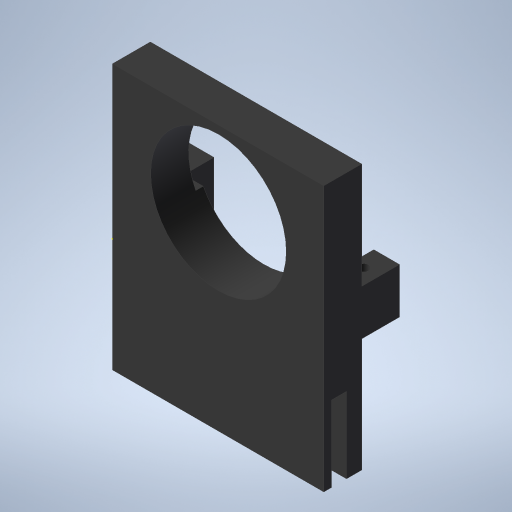
# Autodesk Inventor part: Part8
Saved by Autodesk Inventor 2023.2 (Build 272271030, 271C)
## iProperties
Created: 2024-03-23
Part Number: Part8
Material: Generic
Document SubType Name: Modeling
Designer: ryanv
Density: 1 g/cm^3
Appearance: Default
Author: ryanv
Autodesk Inventor part; units mm, degrees
ref_plane "YZ Plane" through (0, 0, 0) normal (1, 0, 0) x (0, 1, 0)
ref_plane "XZ Plane" through (0, 0, 0) normal (0, 1, 0) x (-1, 0, 0)
ref_plane "XY Plane" through (0, 0, 0) normal (0, 0, 1) x (1, 0, 0)
sketch "Sketch1" plane through (0, 0, 0) normal (0, 0, 1) x (1, 0, 0)
  line L0 (0, 40) -> (55.8, 40)
  line L1 (55.8, 40) -> (55.8, 0)
  line L2 (55.8, 0) -> (0, 0)
  line L3 (0, 0) -> (0, 40)
  dimension "d0" = 55.8
  dimension "d1" = 40
  constraints: 8 end point, 2 parallel, 1 horizontal, 1 perpendicular
  measures "d0" distance of L1.end L2.end
  measures "d1" distance between parallel lines of L2 L0
extrude "Extrusion1" add sketch "Sketch1" along normal blind 20
sketch "Sketch2" plane through (55.8, 0, 0) normal (1, 0, 0) x (0, 0, -1)
  line L0 (0, 40) -> (-20, 40) projected
  line L1 (0, 0) -> (0, 40) projected
  line L2 (-10, 40) -> (0, 40)
  line L3 (0, 40) -> (0, 12)
  line L4 (0, 12) -> (-10, 12)
  line L5 (-10, 12) -> (-10, 40)
  dimension "d4" = 10
  constraints: 8 end point, 2 parallel, 1 horizontal, 1 midpoint, 1 perpendicular, 1 point on line
  measures "d4" distance between parallel lines of L1 L5
extrude "Extrusion2" cut sketch "Sketch2" against normal blind 60
sketch "Sketch3" plane through (55.8, 12, 10) normal (0, 1, 0) x (1, 0, 0)
  circle A0 centre (-51.8, 4.52) radius 1.36
  circle A1 centre (-4, 4.52) radius 1.36
  line L0 (-55.8, 10) -> (0, 10) projected
  line L1 (-55.8, 0) -> (-55.8, 10) projected
  line L2 (0, 10) -> (0, 0) projected
  point P0 (-55.8, 5)
  point P1 (0, 5)
  dimension "d32" = 4
  dimension "d33" = 4
  constraints: 2 centre point, 2 midpoint
  measures "d32" horizontal distance of point (-55.8, 5) A0.centre
  measures "d33" horizontal distance of point (0, 5) A1.centre
extrude "Extrusion3" cut sketch "Sketch3" against normal blind 20
sketch "Sketch4" plane through (0, 0, 20) normal (0, 0, 1) x (1, 0, 0)
  point P0 (0, 0)
sketch "Sketch6" plane through (0, 0, 0) normal (0, 0, -1) x (-1, 0, 0)
  circle A0 centre (-28, 20) radius 17.9
  point P0 (0, 0)
  dimension "d18" = 35.8
  constraints: 1 centre point
  measures "d18" diameter of A0
extrude "Extrusion4" cut sketch "Sketch6" along normal mid plane 60
sketch "Sketch8" plane through (0, 0, 0) normal (0, -1, 0) x (1, 0, 0)
  line L0 (49, 0) -> (6.8, 0)
  line L1 (6.8, 0) -> (6.8, 8)
  line L2 (6.8, 8) -> (49, 8)
  line L3 (49, 8) -> (49, 0)
  line L4 (55.8, 0) -> (55.8, 20) projected
  line L5 (0, 0) -> (0, 20) projected
  point P0 (6.8, 4)
  dimension "d27" = 6.8
  dimension "d28" = 6.8
  constraints: 8 end point, 2 parallel, 1 horizontal, 1 midpoint, 1 perpendicular
  measures "d27" distance between parallel lines of L3 L4
  measures "d28" distance from line of L5 point (6.8, 4)
extrude "Extrusion6" cut sketch "Sketch8" against normal blind 13
sketch "Sketch9" plane through (0, 0, 20) normal (0, -1, 0) x (1, 0, 0)
  line L0 (55.8, 0) -> (0, 0) projected
  line L1 (55.8, -10) -> (55.8, 0) projected
  line L2 (0, 0) -> (55.8, 0)
  line L3 (55.8, 0) -> (55.8, -10)
  line L4 (55.8, -10) -> (0, -10)
  line L5 (0, -10) -> (0, 0)
  point P0 (0, -20)
  dimension "d34" = 10
  constraints: 8 end point, 2 parallel, 1 horizontal, 1 perpendicular, 1 point on line
  measures "d34" distance between parallel lines of L4 L0
extrude "Extrusion7" add sketch "Sketch9" along normal blind 30
sketch "Sketch10" plane through (0, -30, 20) normal (0, -1, 0) x (1, 0, 0)
  line L0 (0, -10) -> (0, 0) projected
  line L1 (55.8, -10) -> (55.8, 0) projected
  line L2 (0, -2) -> (55.8, -2)
  line L3 (55.8, -2) -> (55.8, -6)
  line L4 (55.8, -6) -> (0, -6)
  line L5 (0, -6) -> (0, -2)
  point P0 (0, -20)
  point P1 (0, -6)
  constraints: 8 end point, 2 parallel, 2 point on line, 1 horizontal, 1 perpendicular
extrude "Extrusion8" cut sketch "Sketch10" against normal blind 20
body "Solid1"
